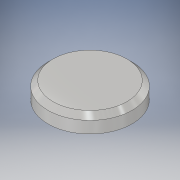
# Autodesk Inventor part: stackLightTop
Saved by Autodesk Inventor 2018 (Build 220112000, 112)
## iProperties
Created: 2017-04-10
Part Number: stackLightTop
Material: ABS Plastic
Document SubType Name: Modeling
Designer: dkt01
Density: 1.06 g/cm^3
Appearance: Aluminum - Polished
Author: dkt01
Autodesk Inventor part; units mm, degrees
ref_plane "YZ Plane" through (0, 0, 0) normal (1, 0, 0) x (0, 1, 0)
ref_plane "XZ Plane" through (0, 0, 0) normal (0, 1, 0) x (-1, 0, 0)
ref_plane "XY Plane" through (0, 0, 0) normal (0, 0, 1) x (1, 0, 0)
sketch "Sketch1" plane through (0, 0, 0) normal (0, 1, 0) x (-1, 0, 0)
  circle A0 centre (0, 0) radius 25
  dimension "d0" = 50
  constraints: 1 centre point, 1 coincident
  measures "d0" diameter of A0
extrude "Extrusion1" add sketch "Sketch1" along normal blind 10
chamfer "Chamfer1" distance 3 angle 45 1 edges at (25, 10, 0)
hole "Hole1" at (0, 0, 0) direction (0, 1, 0) diameter 10 depth 5
body "Solid1"
